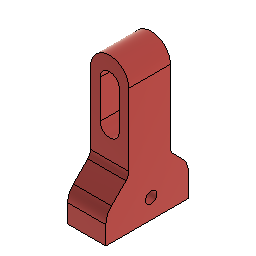
Tower v3 (Autodesk Fusion 360 design; units mm, degrees)
Autodesk Fusion 360 part; units mm, degrees
note: some values were not read from the file. Set by a fixed rule: the direction of a hole.
sketch "Right" plane through (0, 0, 0) normal (1, 0, 0) x (0, 1, 0) in component "Tower"
  line L0 (0, 0) -> (0, 11.6117)
  line L1 (27.432, 9.9611) -> (27.432, 0)
  arc A0 (27.432, 9.9611) -> (25.5721, 14.4512) centre (21.082, 9.9611) ccw
  arc A1 (1.8541, 16.096) -> (0, 11.6117) centre (6.35, 11.6117) ccw
  arc A2 (5.0391, 19.281) -> (5.969, 21.526) centre (2.794, 21.526) ccw
  line L2 (5.0391, 19.281) -> (1.8541, 16.096)
  line L3 (20.7419, 19.2814) -> (25.5721, 14.4512)
  arc A3 (19.812, 21.5265) -> (20.7419, 19.2814) centre (22.987, 21.5265) ccw
  line L4 (19.812, 51.8592) -> (19.812, 21.5265)
  line L5 (19.812, 51.8592) -> (5.969, 51.8592)
  line L6 (5.969, 21.526) -> (5.969, 51.8592)
  line L7 (0, 0) -> (27.432, 0)
  circle A4 centre (12.3596, 10.3275) radius 1.8986
  line L8 (3.937, 0) -> (3.937, 12.7) construction
  line L9 (22.987, 0) -> (22.987, 12.7) construction
  circle A5 centre (12.3596, 10.3275) radius 12.7 construction
  dimension "d1" = 27.432
  dimension "d4" = 10.3275
  dimension "d5" = 6.35
  dimension "d6" = 6.8309
  dimension "d7" = 3.175
  dimension "d8" = 3.175
  dimension "d9" = 6.35
  dimension "d11" = 30.3327
  dimension "d13" = 13.843
  dimension "d14" = 9.9611
  dimension "d16" = 45
  dimension "d17" = 45
  dimension "d19" = 3.937
  dimension "d20" = 19.05
  dimension "d21" = 4.445
  dimension "d22" = 3.7973
  dimension "d23" = 12.3596
  dimension "d24" = 25.5721
  dimension "d25" = 14.4512
  dimension "d26" = 21.5265
  dimension "d28" = 12.7
  dimension "d29" = 12.7
  dimension "d46" = 16.096
  dimension "d47" = 1.8541
  dimension "d48" = 25.4
  constraint tangent A2 L6
  constraint perpendicular L1 L7
  constraint vertical L6
  constraint horizontal L5
  constraint vertical L4
  constraint horizontal L7
  constraint vertical L0
  constraint coincident L0.start L7.start
  constraint coincident L7 L8.start
  constraint perpendicular L7 L8
  constraint coincident L7 L9.start
  constraint perpendicular L7 L9
  constraint tangent A3 L4
  constraint tangent L0 A1
  constraint tangent A2 L2
  constraint concentric A4 A5
  measures "d1" distance of L0.start L1.end
  measures "d4" vertical distance of L0.start A4.centre
  measures "d5" radius of A0
  measures "d6" distance of A0.end L3.start
  measures "d7" radius of A3
  measures "d8" radius of A2
  measures "d9" radius of A1
  measures "d11" distance of A3.start L4.start
  measures "d13" distance of L4.start L5.end
  measures "d14" distance of L1.start L1.end
  measures "d16" angle of L3 L7
  measures "d17" angle of L2 L7
  measures "d19" distance of L0 L8
  measures "d20" distance of L8 L9
  measures "d21" distance of L1 L9
  measures "d22" diameter of A4
  measures "d23" horizontal distance of L0.start A4.centre
  measures "d24" horizontal distance of L0.start A0.end
  measures "d25" vertical distance of L0.start A0.end
  measures "d26" vertical distance of L0.start A3.start
  measures "d28" distance of L8.start L8.end
  measures "d29" distance of L9.start L9.end
  measures "d46" vertical distance of L0.start A1.start
  measures "d47" horizontal distance of L0.start A1.start
  measures "d48" diameter of A5
extrude "Extrude1" add sketch "Right" along normal mid plane 12.7 in component "Tower"
sketch "Front" plane through (0, 0, 0) normal (0, 1, 0) x (1, 0, 0) in component "Tower"
  line L0 (3.175, -43.9217) -> (3.175, -31.2217)
  arc A0 (3.175, -31.2217) -> (-3.175, -31.2217) centre (0, -31.2217) ccw
  line L1 (-3.175, -31.2217) -> (-3.175, -43.9217)
  arc A1 (-3.175, -43.9217) -> (3.175, -43.9217) centre (0, -43.9217) ccw
  line L2 (0, -43.9217) -> (0, -31.2217) construction
  dimension "d32" = 6.35
  dimension "d33" = 31.2217
  dimension "d34" = 12.7
  dimension "d35" = 3.175
  constraint tangent L0 A0
  constraint tangent A0 L1
  constraint parallel L0 L1
  constraint tangent L1 A1
  constraint tangent L0 A1
  constraint vertical L2
  measures "d32" diameter of A0
  measures "d33" vertical distance of A0.centre origin
  measures "d34" distance of A1.centre A0.centre
  measures "d35" horizontal distance of origin A0.end
extrude "Extrude2" cut sketch "Front" along normal up to surface (19.812 mm away) in component "Tower"
sketch "Bottom" plane through (0, 0, 0) normal (0, 0, 1) x (1, 0, 0) in component "Tower"
  circle A0 centre (0, 3.937) radius 1.8986
  circle A1 centre (0, 22.987) radius 1.8986
  dimension "d38" = 19.05
  dimension "d39" = 3.7973
  dimension "d40" = 3.7973
  dimension "d41" = 3.937
  constraint vertical A0.centre origin
  constraint vertical A0.centre A1.centre
  measures "d38" distance of A0.centre A1.centre
  measures "d39" diameter of A1
  measures "d40" diameter of A0
  measures "d41" distance of origin A0.centre
hole "Hole1" at (0, 22.987, 0) at (0, 3.937, 0) direction (0, 0, 1) diameter 3.7973 depth 14.224 tip angle 118 in component "Tower"
fillet "Fillet1" radius 6.35 2 edges at (-6.35, 12.8905, 51.8592) (6.35, 12.8905, 51.8592) in component "Tower"
move_face "OffsetFaces1" offset -3.81 1 faces at (-4.7814, 16.4899, 0) in component "Tower"
component "Tower" placed x (-1, 0, 0) y (0, -1, 0) z (0, 0, 1) at (0, 76.2, 6.8632)
equation "d39 = d40"
